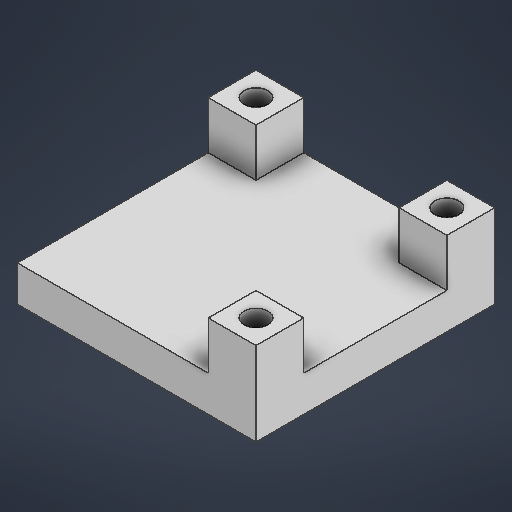
# Autodesk Inventor part: underplate_support_1
Saved by Autodesk Inventor 2026.1 (Build 301233000, 233)
## iProperties
Created: 2025-10-12
Part Number: underplate_support_1
Material: Generic
Document SubType Name: Modeling
Designer: emanuel
Density: 1 g/cm^3
Appearance: Default
Author: emanuel
Autodesk Inventor part; units mm, degrees
ref_plane "YZ Plane" through (0, 0, 0) normal (1, 0, 0) x (0, 1, 0)
ref_plane "XZ Plane" through (0, 0, 0) normal (0, 1, 0) x (-1, 0, 0)
ref_plane "XY Plane" through (0, 0, 0) normal (0, 0, 1) x (1, 0, 0)
sketch "Sketch1" plane through (0, 0, 0) normal (0, 1, 0) x (-1, 0, 0)
  line L0 (0, 0) -> (20, 0)
  line L1 (20, 0) -> (20, -20)
  line L2 (20, -20) -> (0, -20)
  line L3 (0, -20) -> (0, 0)
  dimension "d0" = 20
  dimension "d1" = 20
  constraints: 8 end point, 2 parallel, 1 horizontal, 1 perpendicular
  measures "d0" distance of L1.end L2.end
  measures "d1" distance of L0.end L1.end
extrude "Extrusion1" add sketch "Sketch1" along normal blind 3
sketch "Sketch2" plane through (0, 3, 0) normal (0, 1, 0) x (1, 0, 0)
  line L0 (0, 0) -> (-4, 0)
  line L1 (-4, 0) -> (-4, 4)
  line L2 (-4, 4) -> (0, 4)
  line L3 (0, 4) -> (0, 0)
  line L4 (0, 0) -> (-2, 0)
  line L5 (-2, 0) -> (-2, 2)
  line L6 (-2, 2) -> (0, 2)
  line L7 (0, 2) -> (0, 0)
  line L8 (0, 20) -> (-20, 20) projected
  line L9 (0, 20) -> (-4, 20)
  line L10 (-4, 20) -> (-4, 16)
  line L11 (-4, 16) -> (0, 16)
  line L12 (0, 16) -> (0, 20)
  line L13 (0, 20) -> (-2, 20)
  line L14 (-2, 20) -> (-2, 18)
  line L15 (-2, 18) -> (0, 18)
  line L16 (0, 18) -> (0, 20)
  line L17 (-20, 20) -> (-20, 0) projected
  line L18 (-20, 20) -> (-16, 20)
  line L19 (-16, 20) -> (-16, 16)
  line L20 (-16, 16) -> (-20, 16)
  line L21 (-20, 16) -> (-20, 20)
  line L22 (-20, 20) -> (-18, 20)
  line L23 (-18, 20) -> (-18, 18)
  line L24 (-18, 18) -> (-20, 18)
  line L25 (-20, 18) -> (-20, 20)
  line L26 (-20, 0) -> (-16, 0)
  line L27 (-16, 0) -> (-16, 4)
  line L28 (-16, 4) -> (-20, 4)
  line L29 (-20, 4) -> (-20, 0)
  line L30 (-20, 0) -> (-18, 0)
  line L31 (-18, 0) -> (-18, 2)
  line L32 (-18, 2) -> (-20, 2)
  line L33 (-20, 2) -> (-20, 0)
  circle A0 centre (-18, 2) radius 1
  circle A1 centre (-18, 18) radius 1
  circle A2 centre (-2, 2) radius 1
  circle A3 centre (-2, 18) radius 1
  dimension "d4" = 4
  dimension "d5" = 4
  dimension "d6" = 2
  dimension "d7" = 2
  dimension "d8" = 4
  dimension "d9" = 4
  dimension "d10" = 2
  dimension "d11" = 2
  dimension "d12" = 4
  dimension "d13" = 4
  dimension "d14" = 2
  dimension "d15" = 2
  dimension "d16" = 4
  dimension "d17" = 4
  dimension "d18" = 2
  dimension "d19" = 2
  dimension "d20" = 2
  dimension "d21" = 2
  dimension "d22" = 2
  dimension "d23" = 2
  constraints: 64 end point, 16 parallel, 8 horizontal, 8 perpendicular, 4 centre point, 4 coincident, 2 point on line
  measures "d4" distance of L1.end L2.end
  measures "d5" distance of L0.end L1.end
  measures "d6" distance of L5.end L6.end
  measures "d7" distance of L4.end L5.end
  measures "d8" distance of L11.end L10.end
  measures "d9" distance of L10.end L9.end
  measures "d10" distance of L15.end L14.end
  measures "d11" distance of L14.end L13.end
  measures "d12" distance of L19.end L20.end
  measures "d13" distance of L18.end L19.end
  measures "d14" distance of L23.end L24.end
  measures "d15" distance of L22.end L23.end
  measures "d16" distance of L28.end L27.end
  measures "d17" distance of L27.end L26.end
  measures "d18" distance of L32.end L31.end
  measures "d19" distance of L31.end L30.end
  measures "d20" diameter of A0
  measures "d21" diameter of A1
  measures "d22" diameter of A2
  measures "d23" diameter of A3
extrude "Extrusion2" add sketch "Sketch2" along normal blind 4 contours L0 L5 A2 L6 L3 | L0 L1 L2 L3 L6 A2 L5 | L12 L15 A3 L14 L8 | L19 L20 L17 L24 A1 L23 L8 | L14 A3 L15 L12 L11 L10 L8 | L23 A1 L24 L17 L8
body "Solid1"
